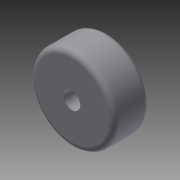
# Autodesk Inventor part: rough pulley
Saved by Autodesk Inventor 2013 (Build 170138000, 138)
## iProperties
Created: 2013-01-20
Part Number: rough pulley
Material: Generic
Document SubType Name: Modeling
Designer: Arpan
Density: 3.8625 g/cm^3
Mass: 136.078 g
Surface Area: 66.1382 cm^2
Volume: 35.2305 cm^3
Author: Arpan
Autodesk Inventor part; units mm, degrees
ref_plane "YZ Plane" through (0, 0, 0) normal (1, 0, 0) x (0, 1, 0)
ref_plane "XZ Plane" through (0, 0, 0) normal (0, 1, 0) x (-1, 0, 0)
ref_plane "XY Plane" through (0, 0, 0) normal (0, 0, 1) x (1, 0, 0)
sketch "Sketch1" plane through (0, 0, 0) normal (0, 0, 1) x (1, 0, 0)
  circle A0 centre (0, 0) radius 23.8125
  dimension "d0" = 47.625
  constraints: 1 centre point, 1 coincident
  measures "d0" diameter of A0
extrude "Extrusion1" add sketch "Sketch1" along normal blind 20.6375
sketch "Sketch2" plane through (0, 0, 20.6375) normal (0, 0, 1) x (1, 0, 0)
  circle A0 centre (0, 0) radius 23.8125 projected
  circle A1 centre (0, 0) radius 4.7625
  dimension "d3" = 9.525
  constraints: 1 centre point, 1 coincident
  measures "d3" diameter of A1
extrude "Extrusion2" cut sketch "Sketch2" against normal blind 12.7 contours A1
fillet "Fillet1" radius 3.175 2 edges at (-23.8125, 0, 20.6375) (-23.8125, 0, 0)
body "Solid1"
